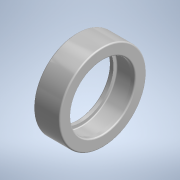
# Autodesk Inventor part: 110202DT-20-L1260ZZ_or
Saved by Autodesk Inventor 2021.3 (Build 253353000, 353)
## iProperties
Part Number: 110202DT-20-L1260ZZ_or
Material: アセタール樹脂、白
Catalog Web Link: www.cadenas.de
Description: DT or-I-Series bearings
Vendor: TOKBEARING
Document SubType Name: Modeling
Designer: partserver
Manufacturer: TOKBEARING
Mass: 0.98693 g
Surface Area: 10.017 cm^2
Volume: 0.692582 cm^3
Density: 1.425 g/cm^3
Appearance: 白
Category: PARTsolutions
Company: TOKBEARING
PSOL_IDENT_0: {$CADENAS_DATA\23d-libs\tok_bearing\i_series_bearings\dt\dt_or.prj},185 {VTYP=3D},{NB=110202DT-20-L1
PSOL_IDENT_1: 260ZZ_or},{LINA=110202DT-20-L1260ZZ_or},{NN=DT or},{DATE=16.12.2020 00:38:07},{GEOMDATE=30.07.2014 0
PSOL_IDENT_2: 8:04:00},{VERSION=},{LINEID=2930},{WBVAR=},{WBNUMERIC=}  {NB=110202DT-20-L1260ZZ_or},{LINA=110202DT-
PSOL_IDENT_3: 20-L1260ZZ_or},{KT=DUMMY},{IDNR=},{CODE=110202},{PN=DT-20-L1260ZZ},{D=20},{SD=6},{SDX=6.000},{W=6},{
PSOL_IDENT_4: C=-},{CX=0.000},{L=-},{LX=0.000},{N=-},{NX=0.000},{TYPE=1},{B=4},{BD=4},{OP=35.168},{BQ=5},{R=5.6},{
PSOL_IDENT_5: GP=2.4}
NB: 110202DT-20-L1260ZZ_or
NN: DT or
NT: I-Series bearings
NBSYN: $CODE.$PN._or
LINA: 110202DT-20-L1260ZZ_or
CATALOG: TOK, Inc
CODE: 110202
PN: DT-20-L1260ZZ
D: 20
SD: 6
SDX: 6
W: 6
C: -
CX: 0
L: -
LX: 0
N: -
NX: 0
TYPE: 1
B: 4
SUPPLIER: TOKBEARING
ARTICLENO: 110202DT-20-L1260ZZ_or
BOMINFO: 110202DT-20-L1260ZZ_or
CREATOR: CADENAS GmbH
Title: 110202DT-20-L1260ZZ_or
Author: Cadenas PARTsolutions
Comments: I-Series bearings
Autodesk Inventor part; units mm, degrees
sketch "Sketch_1" plane through (0, 0, 0) normal (0, 0, 1) x (1, 0, 0)
  line L0 (6, 0) -> (0, 0)
  arc A0 (0, 7.7) -> (0.3, 7.4) centre (0.3, 7.7) ccw
  line L1 (0.3, 7.4) -> (1, 7.4)
  line L2 (1, 7.4) -> (1, 8)
  arc A1 (1.2, 8.2) -> (1, 8) centre (1.2, 8) ccw
  line L3 (1.2, 8.2) -> (4.8, 8.2)
  arc A2 (5, 8) -> (4.8, 8.2) centre (4.8, 8) ccw
  line L4 (5, 8) -> (5, 7.4)
  line L5 (5, 7.4) -> (5.7, 7.4)
  arc A3 (5.7, 7.4) -> (6, 7.7) centre (5.7, 7.7) ccw
  line L6 (6, 7.7) -> (6, 9.7)
  arc A4 (6, 9.7) -> (5.7, 10) centre (5.7, 9.7) ccw
  line L7 (5.7, 10) -> (0.3, 10)
  arc A5 (0.3, 10) -> (0, 9.7) centre (0.3, 9.7) ccw
  line L8 (0, 9.7) -> (0, 7.7)
  constraints: 18 end point, 12 point on circle, 6 centre point
revolve "Revolution1" add sketch "Sketch_1" angle 360 about axis through (6, 0, 0) along (1, 0, 0)
ref_plane "IP_roller_typ1_XY" through (3, 0, 0) normal (1, 0, 0) x (0, 0, -1)
ref_plane "IP_roller_typ1_YZ" through (3, 0, 0) normal (0, 0, -1) x (0, 1, 0)
ref_plane "IP_roller_typ1_ZX" through (3, 0, 0) normal (0, 1, 0) x (1, 0, 0)
ref_plane "OR_IR_XY" through (0, 0, 0) normal (1, 0, 0) x (0, 0, -1)
ref_plane "OR_IR_YZ" through (0, 0, 0) normal (0, 0, -1) x (0, 1, 0)
ref_plane "OR_IR_ZX" through (0, 0, 0) normal (0, 1, 0) x (1, 0, 0)
ref_plane "OR_ball_1_XY" through (3, 5.6, 0) normal (1, 0, 0) x (0, 0, -1)
ref_plane "OR_ball_1_YZ" through (3, 5.6, 0) normal (0, 0, -1) x (0, 1, 0)
ref_plane "OR_ball_1_ZX" through (3, 5.6, 0) normal (0, 1, 0) x (1, 0, 0)
ref_plane "OR_ball_2_XY" through (3, 1.7305, 5.3259) normal (1, 0, 0) x (0, 0, -1)
ref_plane "OR_ball_2_YZ" through (3, 1.7305, 5.3259) normal (0, 0, -1) x (0, 1, 0)
ref_plane "OR_ball_2_ZX" through (3, 1.7305, 5.3259) normal (0, 1, 0) x (1, 0, 0)
ref_plane "OR_ball_3_XY" through (3, -4.5305, 3.2916) normal (1, 0, 0) x (0, 0, -1)
ref_plane "OR_ball_3_YZ" through (3, -4.5305, 3.2916) normal (0, 0, -1) x (0, 1, 0)
ref_plane "OR_ball_3_ZX" through (3, -4.5305, 3.2916) normal (0, 1, 0) x (1, 0, 0)
ref_plane "OR_ball_4_XY" through (3, -4.5305, -3.2916) normal (1, 0, 0) x (0, 0, -1)
ref_plane "OR_ball_4_YZ" through (3, -4.5305, -3.2916) normal (0, 0, -1) x (0, 1, 0)
ref_plane "OR_ball_4_ZX" through (3, -4.5305, -3.2916) normal (0, 1, 0) x (1, 0, 0)
ref_plane "OR_ball_5_XY" through (3, 1.7305, -5.3259) normal (1, 0, 0) x (0, 0, -1)
ref_plane "OR_ball_5_YZ" through (3, 1.7305, -5.3259) normal (0, 0, -1) x (0, 1, 0)
ref_plane "OR_ball_5_ZX" through (3, 1.7305, -5.3259) normal (0, 1, 0) x (1, 0, 0)
ref_plane "OR_dummy_XY" through (0, 0, 0) normal (1, 0, 0) x (0, 0, -1)
ref_plane "OR_dummy_YZ" through (0, 0, 0) normal (0, 0, -1) x (0, 1, 0)
ref_plane "OR_dummy_ZX" through (0, 0, 0) normal (0, 1, 0) x (1, 0, 0)
body "Solid1"
